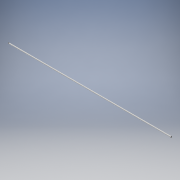
# Autodesk Inventor part: Bottom pipe
Saved by Autodesk Inventor 2017 (Build 210142000, 142)
## iProperties
Created: 2017-11-09
Part Number: Bottom pipe
Material: Generic
Document SubType Name: Modeling
Designer: DesignPC02
Density: 1 g/cm^3
Appearance: Default
Author: DesignPC02
Autodesk Inventor part; units mm, degrees
ref_plane "YZ Plane" through (0, 0, 0) normal (1, 0, 0) x (0, 1, 0)
ref_plane "XZ Plane" through (0, 0, 0) normal (0, 1, 0) x (-1, 0, 0)
ref_plane "XY Plane" through (0, 0, 0) normal (0, 0, 1) x (1, 0, 0)
sketch "Sketch1" plane through (0, 0, 0) normal (1, 0, 0) x (0, 1, 0)
  circle A0 centre (0, 0) radius 13
  circle A1 centre (0, 0) radius 10.3
  dimension "d0" = 26
  dimension "d1" = 2.7
  constraints: 2 centre point, 1 coincident
  measures "d0" diameter of A0
  measures "d1" radial gap between concentric circles of A0 A1
extrude "Extrusion1" add sketch "Sketch1" along normal mid plane 4000
body "Solid1"
